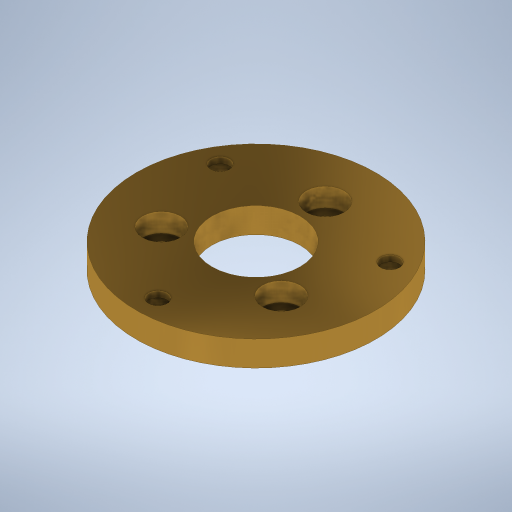
# Autodesk Inventor part: Insert_flange_Top
Saved by Autodesk Inventor 2024 (Build 280153000, 153)
## iProperties
Created: 2023-09-24
Part Number: Insert_flange_Top
Material: Brass
Document SubType Name: Modeling
Designer: schanen
Density: 8.49 g/cm^3
Appearance: Brass - Polished
CD: 15.600 mm
OD: 4.000 mm
WA: 0.300 mm
THR: 3.000 mm
Author: schanen
Autodesk Inventor part; units mm, degrees
ref_plane "YZ Plane" through (0, 0, 0) normal (1, 0, 0) x (0, 1, 0)
ref_plane "XZ Plane" through (0, 0, 0) normal (0, 1, 0) x (-1, 0, 0)
ref_plane "XY Plane" through (0, 0, 0) normal (0, 0, 1) x (1, 0, 0)
sketch "Sketch1" plane through (0, 0, 0) normal (0, 0, 1) x (1, 0, 0)
  line L0 (-7, 0) -> (-19, 0)
  line L1 (-19, 0) -> (-19, 4)
  line L2 (-19, 4) -> (-7, 4)
  line L3 (-7, 4) -> (-7, 0)
  line L4 (0, -0.8) -> (0, 4.8) projected
  point P0 (0, 0)
  dimension "d0" = 19
  dimension "d1" = 7
  dimension "d2" = 4
  constraints: 8 end point, 2 parallel, 1 horizontal, 1 perpendicular
  measures "d0" distance from line of point (0, 0) L1
  measures "d1" distance from line of point (0, 0) L3
  measures "d2" distance of L0.end L1.end
revolve "Revolution1" add sketch "Sketch1" angle 360 about axis through (0, -10, 0) along (0, 1, 0)
sketch "Sketch3" plane through (0, 4, 0) normal (0, 1, 0) x (1, 0, 0)
  point P0 (0, 0)
  point P1 (0, 11)
  dimension "d16" = 11
  measures "d16" distance of point (0, 0) point (0, 11)
hole "Hole2" at (0, 4, -11) direction (0, -1, 0) diameter 3 end through all counterbore diameter 6 counterbore depth 3
pattern_circular "Circular Pattern1" count 3 over 360 about axis through (0, 2, 0) along (0, 1, 0) of "Hole2"
sketch "Sketch4" plane through (0, 0, 0) normal (0, -1, 0) x (1, 0, 0)
  point P0 (0, 0)
  point P1 (0, 15.6)
  dimension "d27" = 15.6
  measures "d27" distance of point (0, 0) point (0, 15.6)
hole "Hole3" at (0, 0, 15.6) direction (0, 1, 0) diameter 3 end through all counterbore diameter 6 counterbore depth 3
pattern_circular "Circular Pattern2" count 3 over 360 about axis through (0, 2, 0) along (0, 1, 0) of "Hole3"
equation "\"d27\" = CD"
equation "\"CD\" = 15.6"
equation "\"OD\" = 4"
equation "\"WA\" = 0.3"
equation "\"THR\" = 3"
body "Solid1"
